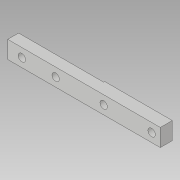
# Autodesk Inventor part: connection_hand_camera
Saved by Autodesk Inventor 2017 (Build 210142000, 142)
## iProperties
Part Number: connection_hand_camera
Material: Generisch
Document SubType Name: Modeling
Designer: Max
Density: 1 g/cm^3
Appearance: Vorgabe
Author: Max
Autodesk Inventor part; units mm, degrees
ref_plane "YZ Plane" through (0, 0, 0) normal (1, 0, 0) x (0, 1, 0)
ref_plane "XZ Plane" through (0, 0, 0) normal (0, 1, 0) x (-1, 0, 0)
ref_plane "XY Plane" through (0, 0, 0) normal (0, 0, 1) x (1, 0, 0)
sketch "Skizze1" plane through (0, 0, 0) normal (0, 1, 0) x (-1, 0, 0)
  line L0 (-35, 4) -> (35, 4)
  line L1 (35, 4) -> (35, -4)
  line L2 (35, -4) -> (-35, -4)
  line L3 (-35, -4) -> (-35, 4)
  line L4 (-35, 4) -> (35, -4) construction
  line L5 (35, 4) -> (-35, -4) construction
  point P0 (0, 0)
  dimension "d0" = 70
  dimension "d1" = 8
  constraints: 12 end point, 2 midpoint, 2 parallel, 1 horizontal, 1 perpendicular
  measures "d0" distance of L1.end L2.end
  measures "d1" distance of L2.end L0.start
extrude "Extrusion1" add sketch "Skizze1" along normal blind 5
sketch "Skizze2" plane through (0, 5, 0) normal (0, 1, 0) x (1, 0, 0)
  line L0 (-35, -4) -> (35, -4) projected
  line L1 (35, -4) -> (35, 4) projected
  line L2 (35, 4) -> (-35, 4) projected
  line L3 (-35, 4) -> (-35, -4) projected
  line L4 (0, 0) -> (47.4069, 0) construction
  point P0 (31, 0)
  point P1 (9, 0)
  dimension "d4" = 8
  dimension "d5" = 4
  dimension "d7" = 22
  constraints: 2 end point, 2 point on line, 1 horizontal
  measures "d4" distance of L0.end L1.end
  measures "d5" distance from line of point (31, 0) L1
  measures "d7" distance of point (31, 0) point (9, 0)
hole "Bohrung1" at (31, 5, 0) at (9, 5, 0) direction (0, -1, 0) diameter 3.4 end through all clearance for "Inbusschraube ISO 4762" size "M3" standard "ISO"
sketch "Skizze3" plane through (0, 5, 0) normal (0, 1, 0) x (1, 0, 0)
  line L0 (19.9613, 0) -> (-27.7601, 0) construction
  circle A0 centre (9, 0) radius 1.7 projected
  point P0 (0, 0)
  point P1 (-13, 0)
  point P2 (-28.5, 0)
  dimension "d15" = 22
  dimension "d16" = 15.5
  constraints: 3 point on line, 2 end point, 1 horizontal
  measures "d15" distance of point (-13, 0) A0.centre
  measures "d16" distance of point (-28.5, 0) point (-13, 0)
hole "Bohrung2" at (-13, 5, 0) at (-28.5, 5, 0) direction (0, -1, 0) diameter 3.4 end through all clearance for "Inbusschraube ISO 4762" size "M3" standard "ISO"
sketch "Skizze4" plane through (0, 5, 0) normal (0, 1, 0) x (1, 0, 0)
  circle A0 centre (-13, 0) radius 1.7 projected
  circle A1 centre (-28.5, 0) radius 1.7 projected
  circle A2 centre (31, 0) radius 1.7 projected
  circle A3 centre (9, 0) radius 1.7 projected
  line L0 (-35, -4) -> (35, -4) projected
  line L1 (35, -4) -> (35, 4) projected
  line L2 (35, 4) -> (-35, 4) projected
  line L3 (-35, 4) -> (-35, -4) projected
  line L4 (-35, 4) -> (35, 4) projected
  line L5 (35, -4) -> (4, -4)
  line L6 (4, -4) -> (4, 4)
  line L7 (4, 4) -> (35, 4)
  line L8 (35, 4) -> (35, -4)
  point P0 (0, 0)
  dimension "d27" = 5
  constraints: 8 end point, 2 parallel, 1 horizontal, 1 perpendicular, 1 point on line
  measures "d27" distance from line of A3.centre L6
extrude "Extrusion2" add sketch "Skizze4" along normal blind 0.5 contours L6 L2 L1 L0
equation "\"d5\" = 0.5 * d4"
